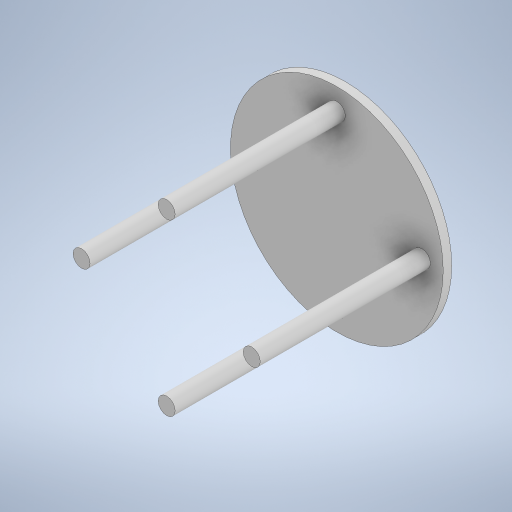
# Autodesk Inventor part: Maitri_table
Saved by Autodesk Inventor 2023 (Build 270158000, 158)
## iProperties
Created: 2023-10-24
Part Number: Maitri_table
Material: Generic
Document SubType Name: Modeling
Designer: maitr
Density: 1 g/cm^3
Appearance: Default
Author: maitr
Autodesk Inventor part; units mm, degrees
ref_plane "YZ Plane" through (0, 0, 0) normal (1, 0, 0) x (0, 1, 0)
ref_plane "XZ Plane" through (0, 0, 0) normal (0, 1, 0) x (-1, 0, 0)
sketch "Sketch1" plane through (0, 0, 0) normal (0, 0, 1) x (1, 0, 0)
  circle A0 centre (0, 0) radius 500
  dimension "d0" = 1000
  constraints: 1 centre point, 1 coincident
  measures "d0" diameter of A0
extrude "Extrusion1" add sketch "Sketch1" along normal blind 40
ref_plane "Work Plane1" through (0, 0, 40) normal (0, 0, 1) x (1, 0, 0)
sketch "Sketch2" plane through (0, 0, 40) normal (0, 0, 1) x (1, 0, 0)
  circle A0 centre (0, 400) radius 40
  circle A1 centre (400, 0) radius 40
  circle A2 centre (0, -400) radius 40
  circle A3 centre (-400, 0) radius 40
  point P0 (0, 0)
  dimension "d4" = 80
  dimension "d5" = 80
  dimension "d6" = 80
  dimension "d7" = 80
  dimension "d8" = 400
  dimension "d9" = 400
  dimension "d10" = 400
  dimension "d11" = 400
  constraints: 4 centre point
  measures "d4" diameter of A0
  measures "d5" diameter of A1
  measures "d6" diameter of A2
  measures "d7" diameter of A3
  measures "d8" distance of A3.centre point (0, 0)
  measures "d9" distance of point (0, 0) A1.centre
  measures "d10" distance of point (0, 0) A0.centre
  measures "d11" distance of A2.centre point (0, 0)
extrude "Extrusion2" add sketch "Sketch2" along normal blind 800
body "Solid1"
